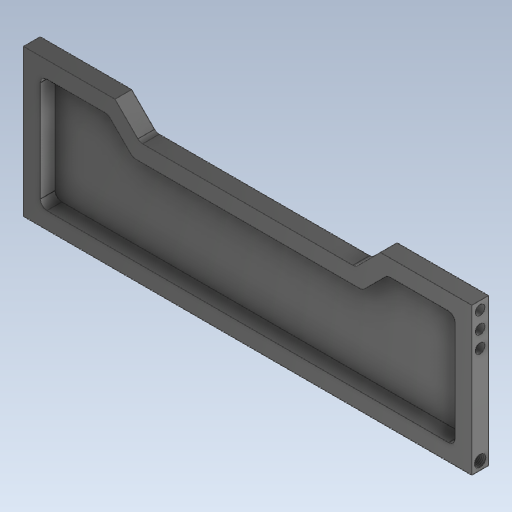
# Autodesk Inventor part: Cockpit_battery_back_door
Saved by Autodesk Inventor 2020 (Build 240168000, 168)
## iProperties
Part Number: Cockpit_battery_back_door
Material: アセタール樹脂、黒
Document SubType Name: Modeling
Designer: Masato Kubotera
Density: 1.425 g/cm^3
Appearance: 滑らか - 黒
Description: POM T5
Mass: 14.6369 g
Surface Area: 144.283 cm^2
Volume: 10.2715 cm^3
Author: Masato Kubotera
Autodesk Inventor part; units mm, degrees
ref_plane "XZ Plane" through (0, 0, 0) normal (0, 1, 0) x (-1, 0, 0)
ref_plane "XY Plane" through (0, 0, 0) normal (0, 0, 1) x (1, 0, 0)
derived "Cockpit_side_frame.ipt"
sketch "スケッチ2" plane through (0, 0, 0) normal (0, 1, 0) x (-1, 0, 0)
  line L0 (-28.5, -22.5) -> (88.5, -22.5) construction
  line L1 (88.5, -22.5) -> (88.5, -138.5)
  line L2 (88.5, -96) -> (-28.5, -96) construction
  line L3 (-28.5, -96) -> (-28.5, -22.5) construction
  line L4 (-28.5, -22.5) -> (88.5, -96) construction
  line L5 (88.5, -22.5) -> (-28.5, -96) construction
  line L6 (38.5, -101) -> (38.5, -133.5)
  line L7 (43.5, -138.5) -> (88.5, -138.5)
  arc A0 (64.6349, -63.15) -> (63.15, -64.6349) centre (63.8925, -63.8925) ccw
  arc A1 (73.15, -65.2849) -> (71.6651, -63.8) centre (72.4075, -64.5425) ccw
  line L8 (65.3349, -63.8) -> (71.6651, -63.8)
  line L9 (64.6349, -63.15) -> (72.3651, -63.15)
  line L10 (63.9, -63.85) -> (73.1, -63.85) construction
  arc A2 (65.3349, -63.8) -> (63.85, -65.2849) centre (64.5925, -64.5425) ccw
  line L11 (63.2, -63.2) -> (73.8, -63.2) construction
  line L12 (73.15, -65.2849) -> (73.15, -76.2151)
  line L13 (73.8, -70.75) -> (63.2, -70.75) construction
  line L14 (73.85, -64.6349) -> (73.85, -76.8651)
  line L15 (73.1, -63.85) -> (73.1, -77.65) construction
  line L16 (63.85, -65.2849) -> (63.85, -76.2151)
  line L17 (73.8, -63.2) -> (73.8, -78.3) construction
  line L18 (63.15, -64.6349) -> (63.15, -76.8651)
  line L19 (68.5, -63.2) -> (68.5, -78.3) construction
  line L20 (63.9, -77.65) -> (63.9, -63.85) construction
  line L21 (73.1, -63.85) -> (63.9, -77.65) construction
  line L22 (73.8, -63.2) -> (63.2, -78.3) construction
  line L23 (63.2, -63.2) -> (73.8, -78.3) construction
  line L24 (63.2, -78.3) -> (63.2, -63.2) construction
  line L25 (63.9, -63.85) -> (73.1, -77.65) construction
  arc A3 (73.85, -64.6349) -> (72.3651, -63.15) centre (73.1075, -63.8925) ccw
  line L26 (73.1, -77.65) -> (63.9, -77.65) construction
  line L27 (73.8, -78.3) -> (63.2, -78.3) construction
  arc A4 (63.85, -76.2151) -> (65.3349, -77.7) centre (64.5925, -76.9575) ccw
  arc A5 (63.15, -76.8651) -> (64.6349, -78.35) centre (63.8925, -77.6075) ccw
  line L28 (65.3349, -77.7) -> (71.6651, -77.7)
  line L29 (64.6349, -78.35) -> (72.3651, -78.35)
  arc A6 (71.6651, -77.7) -> (73.15, -76.2151) centre (72.4075, -76.9575) ccw
  arc A7 (72.3651, -78.35) -> (73.85, -76.8651) centre (73.1075, -77.6075) ccw
  line L30 (-23.5, -22.5) -> (-28.5, -27.5)
  line L31 (-28.5, -59.25) -> (88.5, -59.25) construction
  line L32 (30, -22.5) -> (30, -96) construction
  line L33 (-23.5, -96) -> (-28.5, -91)
  line L34 (-28.5, -27.5) -> (-28.5, -91)
  line L35 (-20.5, -24.5) -> (-25.5, -24.5) construction
  line L36 (-25.5, -24.5) -> (-25.5, -94) construction
  line L37 (-25.5, -94) -> (-20.5, -94) construction
  line L38 (-20.5, -94) -> (-20.5, -24.5) construction
  line L39 (-20.5, -24.5) -> (-25.5, -94) construction
  line L40 (-25.5, -24.5) -> (-20.5, -94) construction
  line L41 (-25.55, -46.7) -> (-20.45, -46.7)
  line L42 (-20.45, -46.7) -> (-20.45, -71.8)
  line L43 (-20.45, -71.8) -> (-25.55, -71.8)
  line L44 (-25.55, -71.8) -> (-25.55, -46.7)
  line L45 (-25.55, -46.7) -> (-20.45, -71.8) construction
  line L46 (-20.45, -46.7) -> (-25.55, -71.8) construction
  line L47 (-25.5, -46.75) -> (-20.5, -46.75) construction
  line L48 (-25.5, -71.75) -> (-20.5, -71.75) construction
  line L49 (-23, -24.5) -> (-23, -94) construction
  circle A8 centre (-23, -35) radius 3
  circle A9 centre (-23, -35) radius 1.6
  arc A10 (-24.0651, -46.7) -> (-25.55, -48.1849) centre (-24.8075, -47.4425) ccw
  arc A11 (-20.45, -48.1849) -> (-21.9349, -46.7) centre (-21.1925, -47.4425) ccw
  arc A12 (-21.9349, -71.8) -> (-20.45, -70.3151) centre (-21.1925, -71.0575) ccw
  arc A13 (-25.55, -70.3151) -> (-24.0651, -71.8) centre (-24.8075, -71.0575) ccw
  circle A14 centre (-23, -83.5) radius 1.6
  circle A15 centre (-23, -83.5) radius 3
  line L50 (33.5, -96) -> (38.5, -101)
  line L51 (-23.5, -96) -> (33.5, -96)
  line L52 (81, -42.5) -> (-20.5, -42.5) construction
  line L53 (-20.5, -42.5) -> (-20.5, -37.5) construction
  line L54 (-20.5, -37.5) -> (81, -37.5) construction
  line L55 (81, -37.5) -> (81, -42.5) construction
  line L56 (81, -42.5) -> (-20.5, -37.5) construction
  line L57 (-20.5, -42.5) -> (81, -37.5) construction
  line L58 (-20.5, -40) -> (81, -40) construction
  line L59 (30.25, -37.5) -> (30.25, -42.5) construction
  line L60 (5.25, -37.5) -> (5.25, -42.5) construction
  line L61 (55.3, -37.45) -> (5.2, -37.45)
  line L62 (5.2, -37.45) -> (5.2, -42.55)
  line L63 (5.2, -42.55) -> (55.3, -42.55)
  line L64 (55.3, -42.55) -> (55.3, -37.45)
  line L65 (55.3, -37.45) -> (5.2, -42.55) construction
  line L66 (5.2, -37.45) -> (55.3, -42.55) construction
  arc A16 (6.6849, -37.45) -> (5.2, -38.9349) centre (5.9425, -38.1925) ccw
  circle A17 centre (-2.25, -40) radius 3
  circle A18 centre (-2.25, -40) radius 1.6
  line L67 (55.25, -37.5) -> (55.25, -42.5) construction
  arc A19 (55.3, -38.9349) -> (53.8151, -37.45) centre (54.5575, -38.1925) ccw
  circle A20 centre (62.75, -40) radius 3
  circle A21 centre (62.75, -40) radius 1.6
  arc A22 (5.2, -41.0651) -> (6.6849, -42.55) centre (5.9425, -41.8075) ccw
  arc A23 (53.8151, -42.55) -> (55.3, -41.0651) centre (54.5575, -41.8075) ccw
  line L68 (-20.5, -89) -> (81, -89) construction
  line L69 (81, -89) -> (81, -94) construction
  line L70 (81, -94) -> (-20.5, -94) construction
  line L71 (-20.5, -94) -> (-20.5, -89) construction
  line L72 (-20.5, -89) -> (81, -94) construction
  line L73 (81, -89) -> (-20.5, -94) construction
  line L74 (-20.5, -91.5) -> (81, -91.5) construction
  line L75 (30.25, -89) -> (30.25, -94) construction
  line L76 (55.3, -91.55) -> (5.2, -91.55)
  line L77 (5.2, -91.55) -> (5.2, -88.95)
  line L78 (5.2, -88.95) -> (55.3, -88.95)
  line L79 (55.3, -88.95) -> (55.3, -91.55)
  line L80 (55.3, -91.55) -> (5.2, -88.95) construction
  line L81 (5.2, -91.55) -> (55.3, -88.95) construction
  line L82 (5.25, -89) -> (5.25, -91.5) construction
  line L83 (55.25, -89) -> (55.25, -91.5) construction
  line L84 (5.25, -90.25) -> (55.25, -90.25) construction
  arc A24 (7.3, -88.95) -> (5.2, -88.95) centre (6.25, -88.95) ccw
  arc A25 (55.3, -88.95) -> (53.2, -88.95) centre (54.25, -88.95) ccw
  arc A26 (53.2, -91.55) -> (55.3, -91.55) centre (54.25, -91.55) ccw
  arc A27 (5.2, -91.55) -> (7.3, -91.55) centre (6.25, -91.55) ccw
  circle A28 centre (-2.5, -91.5) radius 3
  circle A29 centre (-2.5, -91.5) radius 1.6
  circle A30 centre (62.5, -91.5) radius 3 construction
  circle A31 centre (62.5, -91.5) radius 1.6 construction
  line L85 (-23.5, -22.5) -> (63.7651, -22.5)
  line L86 (65.25, -21.0151) -> (65.25, -17.5)
  line L87 (65.25, -17.5) -> (73.25, -17.5)
  line L88 (73.25, -17.5) -> (73.25, -21.0151)
  line L89 (81, -22.5) -> (81, -17.5)
  line L90 (88.5, -22.5) -> (88.5, -20)
  line L91 (81, -17.5) -> (86, -17.5)
  line L92 (86, -17.5) -> (88.5, -20)
  line L93 (69.25, -17.5) -> (69.25, -22.5) construction
  arc A32 (63.7651, -22.5) -> (65.25, -21.0151) centre (64.5075, -21.7575) ccw
  arc A33 (73.25, -21.0151) -> (74.7349, -22.5) centre (73.9925, -21.7575) ccw
  arc A34 (79.5151, -22.5) -> (81, -21.0151) centre (80.2575, -21.7575) ccw
  line L94 (-15.5, -89) -> (-15.5, -69) construction
  line L95 (-15.5, -69) -> (64.5, -69) construction
  line L96 (64.5, -69) -> (64.5, -89) construction
  line L97 (45.5, -84) -> (-16.5, -84)
  line L98 (-18.5, -82) -> (-18.5, -63.3955)
  line L99 (-16.5, -61.3955) -> (45.5, -61.3955)
  line L100 (47.5, -63.3955) -> (47.5, -82)
  line L101 (47.5, -84) -> (-18.5, -61.3955) construction
  line L102 (-18.5, -84) -> (47.5, -61.3955) construction
  arc A35 (-16.5, -61.3955) -> (-18.5, -63.3955) centre (-16.5, -63.3955) ccw
  arc A36 (-18.5, -82) -> (-16.5, -84) centre (-16.5, -82) ccw
  arc A37 (45.5, -84) -> (47.5, -82) centre (45.5, -82) ccw
  arc A38 (47.5, -63.3955) -> (45.5, -61.3955) centre (45.5, -63.3955) ccw
  line L103 (38.5, -133.5) -> (43.5, -138.5)
  line L104 (46, -131) -> (41, -131) construction
  line L105 (41, -131) -> (41, -96) construction
  line L106 (41, -96) -> (46, -96) construction
  line L107 (46, -96) -> (46, -131) construction
  line L108 (46, -131) -> (41, -96) construction
  line L109 (41, -131) -> (46, -96) construction
  line L110 (43.5, -96) -> (43.5, -131) construction
  line L111 (41, -113.5) -> (46, -113.5) construction
  line L112 (43.5, -107.5) -> (46, -107.5) construction
  line L113 (43.45, -107.45) -> (46.05, -107.45)
  line L114 (46.05, -107.45) -> (46.05, -119.55)
  line L115 (46.05, -119.55) -> (43.45, -119.55)
  line L116 (43.45, -119.55) -> (43.45, -107.45)
  line L117 (43.45, -107.45) -> (46.05, -119.55) construction
  line L118 (46.05, -107.45) -> (43.45, -119.55) construction
  arc A39 (46.05, -109.55) -> (46.05, -107.45) centre (46.05, -108.5) ccw
  arc A40 (44.9349, -107.45) -> (43.45, -108.9349) centre (44.1925, -108.1925) ccw
  arc A41 (46.05, -119.55) -> (46.05, -117.45) centre (46.05, -118.5) ccw
  line L119 (43.5, -119.5) -> (46, -119.5) construction
  arc A42 (43.45, -118.0651) -> (44.9349, -119.55) centre (44.1925, -118.8075) ccw
  line L120 (44.75, -107.5) -> (44.75, -119.5) construction
  circle A43 centre (43.5, -125.5) radius 3 construction
  circle A44 centre (43.5, -125.5) radius 1.6 construction
  circle A45 centre (43.5, -101.5) radius 3
  circle A46 centre (43.5, -101.5) radius 1.6
  circle A47 centre (-13.5, -55) radius 2
  line L121 (41, -131) -> (79.8645, -131) construction
  line L122 (79.8645, -131) -> (79.8645, -136) construction
  line L123 (79.8645, -136) -> (41, -136) construction
  line L124 (41, -136) -> (41, -131) construction
  line L125 (41, -131) -> (79.8645, -136) construction
  line L126 (79.8645, -131) -> (41, -136) construction
  line L127 (41, -133.5) -> (79.8645, -133.5) construction
  line L128 (60.4322, -131) -> (60.4322, -136) construction
  line L129 (60.4322, -133.5) -> (60.4322, -131) construction
  line L130 (52.8822, -130.95) -> (67.9822, -130.95)
  line L131 (67.9822, -130.95) -> (67.9822, -133.55)
  line L132 (67.9822, -133.55) -> (52.8822, -133.55)
  line L133 (52.8822, -133.55) -> (52.8822, -130.95)
  line L134 (52.8822, -130.95) -> (67.9822, -133.55) construction
  line L135 (67.9822, -130.95) -> (52.8822, -133.55) construction
  line L136 (52.9322, -131) -> (52.9322, -133.5) construction
  arc A48 (54.9822, -130.95) -> (52.8822, -130.95) centre (53.9322, -130.95) ccw
  arc A49 (52.8822, -132.0651) -> (54.3672, -133.55) centre (53.6247, -132.8075) ccw
  arc A50 (67.9822, -130.95) -> (65.8822, -130.95) centre (66.9322, -130.95) ccw
  arc A51 (66.4973, -133.55) -> (67.9822, -132.0651) centre (67.2398, -132.8075) ccw
  line L137 (67.9322, -131) -> (67.9322, -133.5) construction
  line L138 (52.9322, -132.25) -> (67.9322, -132.25) construction
  circle A52 centre (74.4322, -133.5) radius 1.6 construction
  circle A53 centre (74.4322, -133.5) radius 3 construction
  circle A54 centre (46.4322, -133.5) radius 3
  circle A55 centre (46.4322, -133.5) radius 1.6
  line L139 (50.5, -96.5) -> (79, -96.5)
  line L140 (81, -98.5) -> (81, -126.5)
  line L141 (79, -128.5) -> (50.5, -128.5)
  line L142 (48.5, -126.5) -> (48.5, -98.5)
  line L143 (48.5, -96.5) -> (81, -128.5) construction
  line L144 (81, -96.5) -> (48.5, -128.5) construction
  arc A56 (50.5, -96.5) -> (48.5, -98.5) centre (50.5, -98.5) ccw
  arc A57 (48.5, -126.5) -> (50.5, -128.5) centre (50.5, -126.5) ccw
  arc A58 (79, -128.5) -> (81, -126.5) centre (79, -126.5) ccw
  arc A59 (81, -98.5) -> (79, -96.5) centre (79, -98.5) ccw
  line L145 (81, -91.6746) -> (86, -91.6746) construction
  line L146 (86, -91.6746) -> (86, -136) construction
  line L147 (86, -136) -> (81, -136) construction
  line L148 (81, -136) -> (81, -91.6746) construction
  line L149 (81, -91.6746) -> (86, -136) construction
  line L150 (86, -91.6746) -> (81, -136) construction
  line L151 (83.5, -91.6746) -> (83.5, -136) construction
  circle A60 centre (83.5, -94.1746) radius 1.475
  circle A61 centre (83.5, -99.1746) radius 1.475
  circle A62 centre (83.5, -104.1746) radius 1.475
  circle A63 centre (83.5, -133.5) radius 1.6
  arc A64 (86, -91.6746) -> (81, -91.6746) centre (83.5, -133.5) ccw construction
  arc A65 (86.0112, -91.5751) -> (80.9888, -91.5751) centre (83.5, -133.5) ccw construction
  line L152 (88.5, -133.5) -> (83.5, -138.5)
  arc A66 (81, -131) -> (86, -136) centre (83.5, -133.5) ccw construction
  line L153 (86, -91.5) -> (81, -91.5) construction
  circle A67 centre (83.5, -133.5) radius 3
  line L154 (77.125, -22.5) -> (77.125, -27.147) construction
  line L155 (61.375, -22.5) -> (61.375, -27.147) construction
  line L156 (65.25, -22.5) -> (73.25, -22.5)
  line L157 (-18.5, -29.5) -> (-18.5, -31.2215)
  line L158 (-16.5, -33.2215) -> (45.5, -33.2215)
  line L159 (47.5, -31.2215) -> (47.5, -29.5)
  line L160 (45.5, -27.5) -> (-16.5, -27.5)
  arc A68 (-16.5, -27.5) -> (-18.5, -29.5) centre (-16.5, -29.5) ccw
  arc A69 (-18.5, -31.2215) -> (-16.5, -33.2215) centre (-16.5, -31.2215) ccw
  arc A70 (45.5, -33.2215) -> (47.5, -31.2215) centre (45.5, -31.2215) ccw
  arc A71 (47.5, -29.5) -> (45.5, -27.5) centre (45.5, -29.5) ccw
  line L161 (81, -66.9105) -> (86, -66.9105) construction
  line L162 (86, -66.9105) -> (86, -46.9105) construction
  line L163 (86, -46.9105) -> (81, -46.9105) construction
  line L164 (81, -46.9105) -> (81, -66.9105) construction
  line L165 (81, -66.9105) -> (86, -46.9105) construction
  line L166 (86, -66.9105) -> (81, -46.9105) construction
  line L167 (81, -22.5) -> (81, -28.5) construction
  line L168 (81, -28.5) -> (57.5, -28.5) construction
  line L169 (57.5, -28.5) -> (57.5, -22.5) construction
  line L170 (74.7349, -22.5) -> (79.5151, -22.5) construction
  line L171 (74.7349, -22.5) -> (79.5151, -22.5)
  point P0 (0, 0)
  point P1 (30, -59.25)
  point P2 (-25.7227, -96)
  point P3 (63.85, -63.8)
  point P4 (63.15, -63.15)
  point P5 (68.5, -70.75)
  point P6 (-23, -59.25)
  point P7 (30.25, -40)
  point P8 (30.25, -91.5)
  point P9 (30.25, -90.25)
  point P10 (30.25, -90.25)
  point P11 (52.5, -22)
  point P12 (14.5, -72.6978)
  point P13 (-18.5, -61)
  point P14 (47.5, -61)
  point P15 (43.5, -113.5)
  point P16 (44.75, -113.5)
  point P17 (60.4322, -132.25)
  point P18 (64.75, -112.5)
  point P19 (83.5, -113.8373)
  point P20 (-18.5, -33.2215)
  point P21 (47.5, -27.5)
  point P22 (-18.5, -27.5)
  point P23 (73.7349, -22.5)
  point P24 (72.25, -21.0151)
  point P25 (64.4973, -133.55)
  point P26 (63.8822, -130.95)
  point P27 (65.9822, -132.0651)
  point P28 (41.45, -118.0651)
  point P29 (44.05, -117.45)
  point P30 (42.9349, -119.55)
  point P31 (-26.05, -70.3151)
  point P32 (-22.4349, -46.7)
  point P33 (-20.95, -48.1849)
  point P34 (-20.95, -70.3151)
  point P35 (-22.4349, -71.8)
  point P36 (-24.5651, -71.8)
  point P37 (54.05, -59.5651)
  point P38 (52.5651, -61.05)
  point P39 (5.4349, -61.05)
  point P40 (3.95, -59.5651)
  point P41 (52.5651, -55.95)
  point P42 (54.05, -57.4349)
  point P43 (51.95, -88.45)
  point P44 (51.95, -91.05)
  point P45 (6.05, -91.05)
  point P46 (80.4349, -79.8)
  point P47 (78.95, -78.3151)
  point P48 (72.25, -22.5)
  point P49 (83.5, -56.9105)
  point P50 (69.25, -28.5)
  point P51 (73.25, -21.0151)
  point P52 (66.4973, -133.55)
  point P53 (43.45, -118.0651)
  point P54 (44.9349, -119.55)
  point P55 (-25.55, -70.3151)
  point P56 (-21.9349, -46.7)
  point P57 (-21.9349, -71.8)
  point P58 (-24.0651, -71.8)
  point P59 (55.3, -41.0651)
  point P60 (53.8151, -42.55)
  point P61 (6.6849, -42.55)
  point P62 (5.2, -41.0651)
  point P63 (53.8151, -37.45)
  point P64 (55.3, -38.9349)
  point P65 (53.2, -88.95)
  point P66 (53.2, -91.55)
  dimension "d2" = 81
  dimension "d3" = 44.3254
  dimension "d4" = 5
  measures "d2" horizontal distance of L147.end point (0, 0)
  measures "d3" distance of L145.end L146.end
  measures "d4" distance of L146.end L147.end
ref_plane "作業平面1" through (-81, 0, 0) normal (1, 0, 0) x (0, 1, 0)
sketch "スケッチ3" plane through (-81, 0, 0) normal (1, 0, 0) x (0, 1, 0)
  line L0 (-135, -136) -> (0, -136)
  line L1 (0, -136) -> (0, -91.6746)
  line L2 (0, -91.6746) -> (-135, -91.6746)
  line L3 (-135, -91.6746) -> (-135, -136)
  line L4 (-135, -136) -> (0, -91.6746) construction
  line L5 (0, -136) -> (-135, -91.6746) construction
  line L6 (-27.5, -91.6746) -> (-34.4142, -98.5889)
  line L7 (-35.8284, -99.1746) -> (-99.1716, -99.1746)
  line L8 (-100.5858, -98.5889) -> (-107.5, -91.6746)
  line L9 (-67.5, -91.6746) -> (-67.5, -136)
  line L10 (-24.6005, -96.6746) -> (-7, -96.6746)
  line L11 (-5, -98.6746) -> (-5, -129)
  line L12 (-7, -131) -> (-128, -131)
  line L13 (-130, -129) -> (-130, -98.6746)
  line L14 (-128, -96.6746) -> (-110.3995, -96.6746)
  line L15 (-108.9853, -97.2604) -> (-102.6569, -103.5889)
  line L16 (-101.2426, -104.1746) -> (-33.7574, -104.1746)
  line L17 (-32.3431, -103.5889) -> (-26.0147, -97.2604)
  line L18 (0, -113.8373) -> (-135, -113.8373) construction
  arc A0 (-5, -98.6746) -> (-7, -96.6746) centre (-7, -98.6746) ccw
  arc A1 (-24.6005, -96.6746) -> (-26.0147, -97.2604) centre (-24.6005, -98.6746) ccw
  arc A2 (-33.7574, -104.1746) -> (-32.3431, -103.5889) centre (-33.7574, -102.1746) ccw
  arc A3 (-102.6569, -103.5889) -> (-101.2426, -104.1746) centre (-101.2426, -102.1746) ccw
  arc A4 (-108.9853, -97.2604) -> (-110.3995, -96.6746) centre (-110.3995, -98.6746) ccw
  arc A5 (-128, -96.6746) -> (-130, -98.6746) centre (-128, -98.6746) ccw
  arc A6 (-130, -129) -> (-128, -131) centre (-128, -129) ccw
  arc A7 (-7, -131) -> (-5, -129) centre (-7, -129) ccw
  arc A8 (-35.8284, -99.1746) -> (-34.4142, -98.5889) centre (-35.8284, -97.1746) ccw
  arc A9 (-100.5858, -98.5889) -> (-99.1716, -99.1746) centre (-99.1716, -97.1746) ccw
  point P0 (0, 0)
  point P1 (-67.5, -113.8373)
  point P2 (0, -136)
  point P3 (0, -136)
  point P4 (0, -136)
  point P5 (-35, -99.1746)
  point P6 (-5, -96.6746)
  point P7 (-5, -131)
  point P8 (-130, -96.6746)
  point P9 (-109.5711, -96.6746)
  point P10 (-32.9289, -104.1746)
  point P11 (-25.4289, -96.6746)
  point P12 (-67.5, -99.1746)
  point P13 (-67.5, -104.1746)
  point P14 (-67.5, -131)
  dimension "d6" = 135
  dimension "d7" = 5
  dimension "d8" = 5
  dimension "d9" = 7.5
  dimension "d10" = 5
  dimension "d11" = 5
  dimension "d12" = 45
  dimension "d13" = 80
  dimension "d32" = 2
  constraints: 38 end point, 20 point on circle, 20 tangent, 19 point on line, 10 centre point, 9 equal radius, 6 midpoint, 4 parallel, 4 perpendicular, 3 horizontal, 2 coincident, 4 other
  measures "d6" distance of L1.end L2.end
  measures "d7" horizontal distance of L1.end point (-5, -96.675)
  measures "d8" horizontal distance of point (-5, -96.675) L1.end
  measures "d9" distance between parallel lines of L7 L2
  measures "d10" distance between parallel lines of L16 L7
  measures "d11" distance between parallel lines of L17 L6
  measures "d12" angle of L2 L6
  measures "d13" distance of L8.end L6.start
  measures "d32" radius of A0
extrude "押し出し1" add sketch "スケッチ3" against normal blind 5 contours L9 L12 A7 L11 A0 L10 A1 L17 A2 L16 L7 A8 L6 L2 L1 L0 | L9 L16 A2 L17 A1 L10 A0 L11 A7 L12
extrude "押し出し2" cut sketch "スケッチ3" against normal blind 4.5 contours L12 A6 L13 A5 L14 A4 L15 A3 L16 L9 | L9 L16 A2 L17 A1 L10 A0 L11 A7 L12
hole "穴1" at (-83.5, 0, -94.1746) at (-83.5, 0, -99.1746) at (-83.5, 0, -104.1746) direction (0, -1, 0) diameter 2.9 depth 3 tip angle 118
hole "穴2" at (-83.5, 0, -133.5) direction (0, -1, 0) diameter 3.4587 depth 5 thread size "M4x0.5" class "6H" standard "ISO Metric profile"
mirror "ミラー1" about plane through (-81, -67.5, -136) normal (0, -1, 0)
equation "\"d8\" = d7"
equation "\"d10\" = d7"
equation "\"d11\" = d7"
equation "\"d14\" = d4"
equation "\"d1\" = -d2"
